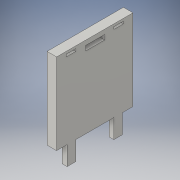
# Autodesk Inventor part: back
Saved by Autodesk Inventor 2016 (Build 200138000, 138)
## iProperties
Created: 2016-08-07
Part Number: back
Material: LCP Plastic
Document SubType Name: Modeling
Designer: Jorian Brusind
Density: 1.626 g/cm^3
Appearance: Smooth - White
Author: Jorian Brusind
Autodesk Inventor part; units mm, degrees
ref_plane "YZ Plane" through (0, 0, 0) normal (1, 0, 0) x (0, 1, 0)
ref_plane "XZ Plane" through (0, 0, 0) normal (0, 1, 0) x (-1, 0, 0)
ref_plane "XY Plane" through (0, 0, 0) normal (0, 0, 1) x (1, 0, 0)
sketch "Sketch1" plane through (0, 0, 0) normal (0, 1, 0) x (-1, 0, 0)
  line L0 (0, 0) -> (12.7, 0)
  line L1 (12.7, 0) -> (12.7, -101.6)
  line L2 (12.7, -101.6) -> (0, -101.6)
  line L3 (0, -101.6) -> (0, 0)
  dimension "d1" = 12.7
  dimension "d2" = 101.6
  constraints: 8 end point, 2 parallel, 1 horizontal, 1 perpendicular
  measures "d1" distance of L1.end L2.end
  measures "d2" distance of L0.end L1.end
extrude "Extrusion1" add sketch "Sketch1" along normal blind 107.95
sketch "Sketch2" plane through (0, 0, 0) normal (0, -1, 0) x (1, 0, 0)
  line L0 (0, 0) -> (0, -101.6) projected
  line L1 (0, -101.6) -> (0, -87.63)
  line L2 (0, 0) -> (0, -13.97)
  line L3 (0, -13.97) -> (-6.35, -13.97)
  line L4 (-6.35, -13.97) -> (-6.35, -25.4)
  line L5 (-6.35, -25.4) -> (0, -25.4)
  line L6 (0, -25.4) -> (0, -13.97)
  line L7 (0, -87.63) -> (-6.35, -87.63)
  line L8 (-6.35, -87.63) -> (-6.35, -76.2)
  line L9 (-6.35, -76.2) -> (0, -76.2)
  line L10 (0, -76.2) -> (0, -87.63)
  dimension "d6" = 13.97
  dimension "d9" = 13.97
  dimension "d10" = 6.35
  dimension "d11" = 11.43
  dimension "d12" = 6.35
  dimension "d13" = 11.43
  constraints: 20 end point, 4 parallel, 2 horizontal, 2 perpendicular, 2 point on line
  measures "d6" distance of L0.end L1.end
  measures "d9" distance of L0.start L2.end
  measures "d10" distance of L5.end L4.end
  measures "d11" distance of L4.end L3.end
  measures "d12" distance of L8.end L9.end
  measures "d13" distance of L7.end L8.end
extrude "Extrusion2" add sketch "Sketch2" along normal blind 25.4
sketch "Sketch3" plane through (0, 0, -101.6) normal (1, 0, 0) x (0, 0, -1)
  line L0 (-101.6, 0) -> (-101.6, 107.95) projected
  line L1 (-101.6, 107.95) -> (-76.2, 107.95)
  line L2 (0, 107.95) -> (-101.6, 107.95) projected
  line L3 (-76.2, 107.95) -> (-76.2, 101.6)
  line L4 (-76.2, 101.6) -> (-88.9, 101.6)
  line L5 (-88.9, 101.6) -> (-88.9, 104.775)
  line L6 (-88.9, 104.775) -> (-76.2, 104.775)
  line L7 (-76.2, 104.775) -> (-76.2, 101.6)
  line L8 (0, 107.95) -> (-25.4, 107.95)
  line L9 (-25.4, 107.95) -> (-25.4, 101.6)
  line L10 (-25.4, 101.6) -> (-12.7, 101.6)
  line L11 (-12.7, 101.6) -> (-12.7, 104.775)
  line L12 (-12.7, 104.775) -> (-25.4, 104.775)
  line L13 (-25.4, 104.775) -> (-25.4, 101.6)
  dimension "d17" = 25.4
  dimension "d18" = 6.35
  dimension "d19" = 12.7
  dimension "d20" = 3.175
  dimension "d21" = 25.4
  dimension "d22" = 6.35
  dimension "d23" = 12.7
  dimension "d24" = 3.175
  constraints: 24 end point, 4 parallel, 2 horizontal, 2 perpendicular, 2 point on line, 2 vertical
  measures "d17" distance of L0.end L1.end
  measures "d18" distance of L1.end L3.end
  measures "d19" distance of L5.end L6.end
  measures "d20" distance of L4.end L5.end
  measures "d21" distance of L2.start L8.end
  measures "d22" distance of L8.end L9.end
  measures "d23" distance of L12.end L11.end
  measures "d24" distance of L11.end L10.end
extrude "Extrusion3" cut sketch "Sketch3" against normal blind 12.7
sketch "Sketch4" plane through (0, 0, -101.6) normal (1, 0, 0) x (0, 0, -1)
  line L0 (-75.6651, 101.8589) -> (-75.6651, 95.5089)
  line L1 (-75.6651, 95.5089) -> (-62.9651, 95.5089)
  line L2 (-62.9651, 95.5089) -> (-37.5651, 95.5089)
  line L3 (-37.5651, 95.5089) -> (-37.5651, 101.8589)
  line L4 (-37.5651, 101.8589) -> (-62.9651, 101.8589)
  line L5 (-62.9651, 101.8589) -> (-62.9651, 95.5089)
  point P0 (-101.6, 0)
  dimension "d29" = 6.35
  dimension "d30" = 12.7
  dimension "d31" = 25.4
  dimension "d32" = 6.35
  constraints: 12 end point, 2 parallel, 2 perpendicular, 1 horizontal, 1 vertical
  measures "d29" distance of L0.start L0.end
  measures "d30" distance of L0.end L1.end
  measures "d31" distance of L4.end L3.end
  measures "d32" distance of L3.end L2.end
extrude "Extrusion4" cut sketch "Sketch4" against normal blind 12.7
body "Solid1"
